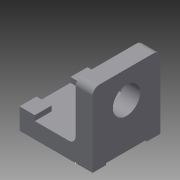
# Autodesk Inventor part: HW 4 Part 2
Saved by Autodesk Inventor 2015 SP1 (Build 190203100, 203)
## iProperties
Created: 2016-01-25
Part Number: HW 4 Part 2
Material: Generic
Document SubType Name: Modeling
Designer: melissa.roth
Density: 1 g/cm^3
Appearance: Default
Author: melissa.roth
Autodesk Inventor part; units mm, degrees
ref_plane "YZ Plane" through (0, 0, 0) normal (1, 0, 0) x (0, 1, 0)
ref_plane "XZ Plane" through (0, 0, 0) normal (0, 1, 0) x (-1, 0, 0)
ref_plane "XY Plane" through (0, 0, 0) normal (0, 0, 1) x (1, 0, 0)
sketch "Sketch1" plane through (0, 0, 0) normal (0, 0, 1) x (1, 0, 0)
  line L0 (0, 0) -> (136.525, 0)
  line L1 (136.525, 0) -> (136.525, 136.525)
  line L2 (136.525, 136.525) -> (104.775, 136.525)
  line L3 (104.775, 136.525) -> (104.775, 42.545)
  line L4 (92.075, 29.845) -> (28.575, 29.845)
  line L5 (28.575, 29.845) -> (28.575, 39.37)
  line L6 (28.575, 39.37) -> (0, 39.37)
  line L7 (0, 39.37) -> (0, 0)
  arc A0 (92.075, 29.845) -> (104.775, 42.545) centre (92.075, 42.545) ccw
  point P0 (104.775, 29.845)
  dimension "d0" = 136.525
  dimension "d1" = 136.525
  dimension "d2" = 31.75
  dimension "d3" = 9.525
  dimension "d4" = 39.37
  dimension "d5" = 76.2
  dimension "d17" = 12.7
  constraints: 16 end point, 5 perpendicular, 2 point on circle, 2 point on line, 2 tangent, 1 centre point, 1 horizontal, 1 parallel, 1 vertical
  measures "d0" distance of L0.start L0.end
  measures "d1" distance of L0.end L1.end
  measures "d2" distance of L1.end L2.end
  measures "d3" distance of L4.end L5.end
  measures "d4" distance of L6.end L0.start
  measures "d5" distance of point (104.775, 29.845) L4.end
  measures "d17" radius of A0
extrude "Extrusion1" add sketch "Sketch1" against normal blind 127
sketch "Sketch2" plane through (0, 39.37, 0) normal (0, 1, 0) x (1, 0, 0)
  line L0 (28.575, 0) -> (28.575, 127) projected
  line L1 (28.575, 95.25) -> (0, 95.25)
  line L2 (0, 95.25) -> (0, 31.75)
  line L3 (0, 0) -> (0, 127) projected
  line L4 (0, 31.75) -> (28.575, 31.75)
  line L5 (0, 127) -> (28.575, 127) projected
  dimension "d9" = 63.5
  dimension "d10" = 31.75
  constraints: 6 end point, 3 point on line, 1 horizontal, 1 perpendicular
  measures "d9" distance of L1.end L2.end
  measures "d10" distance between parallel lines of L5 L1
extrude "Extrusion2" cut sketch "Sketch2" against normal blind 9.525 contours L4 L2 L1 L0
sketch "Sketch3" plane through (0, 0, 0) normal (0, -1, 0) x (1, 0, 0)
  line L0 (0, 0) -> (0, -127) projected
  line L1 (0, -101.6) -> (136.525, -101.6)
  line L2 (136.525, 0) -> (136.525, -127) projected
  line L3 (136.525, -25.4) -> (0, -25.4)
  line L4 (0, 0) -> (136.525, 0) projected
  dimension "d13" = 76.2
  dimension "d14" = 25.4
  constraints: 4 end point, 4 point on line, 1 horizontal, 1 parallel
  measures "d13" distance of L3.start L1.end
  measures "d14" distance between parallel lines of L4 L3
extrude "Extrusion3" cut sketch "Sketch3" against normal blind 3.175 contours L3 L2 L1 L0
sketch "Sketch4" plane through (104.775, 29.845, 0) normal (-1, 0, 0) x (0, 0, 1)
  point P0 (0, -29.845)
sketch "Sketch5" plane through (104.775, 42.545, 0) normal (-1, 0, 0) x (0, 0, 1)
  circle A0 centre (-63.5, 43.18) radius 25.4
  line L0 (-127, 0) -> (-127, 93.98) projected
  line L1 (0, 93.98) -> (-127, 93.98) projected
  point P0 (0, -42.545)
  dimension "d18" = 50.8
  dimension "d19" = 63.5
  dimension "d20" = 50.8
  constraints: 1 centre point
  measures "d18" diameter of A0
  measures "d19" distance from line of L0 A0.centre
  measures "d20" distance from line of L1 A0.centre
extrude "Extrusion4" cut sketch "Sketch5" against normal through all
sketch "Sketch6" plane through (104.775, 42.545, 0) normal (-1, 0, 0) x (0, 0, 1)
  point P0 (0, -42.545)
sketch "Sketch7" plane through (104.775, 42.545, 0) normal (-1, 0, 0) x (0, 0, 1)
  point P0 (0, -42.545)
fillet "Fillet1" radius 12.7 1 edges at (120.65, 136.525, 0)
fillet "Fillet2" radius 12.7 1 edges at (120.65, 136.525, -127)
body "Solid1"
